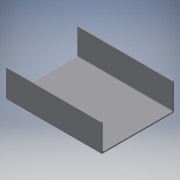
# Autodesk Inventor part: improved lift c chanel
Saved by Autodesk Inventor 2017 (Build 210142000, 142)
## iProperties
Created: 2019-02-04
Part Number: improved lift c chanel
Material: Generic
Document SubType Name: Modeling
Designer: S346852600
Density: 1 g/cm^3
Appearance: Default
Author: S346852600
Autodesk Inventor part; units mm, degrees
ref_plane "YZ Plane" through (0, 0, 0) normal (1, 0, 0) x (0, 1, 0)
ref_plane "XZ Plane" through (0, 0, 0) normal (0, 1, 0) x (-1, 0, 0)
ref_plane "XY Plane" through (0, 0, 0) normal (0, 0, 1) x (1, 0, 0)
sketch "Sketch1" plane through (0, 0, 0) normal (1, 0, 0) x (0, 1, 0)
  line L0 (0, 0) -> (-50.8, 0)
  line L1 (-53.975, -3.175) -> (-53.975, -161.925)
  line L2 (-50.8, -165.1) -> (0, -165.1)
  line L3 (0, -161.925) -> (-47.625, -161.925)
  line L4 (-50.8, -158.75) -> (-50.8, -6.35)
  line L5 (-47.625, -3.175) -> (0, -3.175)
  line L6 (0, 0) -> (0, -3.175)
  line L7 (0, -161.925) -> (0, -165.1)
  arc A0 (-50.8, 0) -> (-53.975, -3.175) centre (-50.8, -3.175) ccw
  arc A1 (-53.975, -161.925) -> (-50.8, -165.1) centre (-50.8, -161.925) ccw
  arc A2 (-47.625, -3.175) -> (-50.8, -6.35) centre (-47.625, -6.35) ccw
  arc A3 (-50.8, -158.75) -> (-47.625, -161.925) centre (-47.625, -158.75) ccw
  point P0 (-50.8, -161.925)
  point P1 (-50.8, -3.175)
  dimension "d3" = 3.175
  dimension "d4" = 50.8
  dimension "d5" = 158.75
  dimension "d6" = 3.175
  constraints: 16 end point, 8 point on circle, 8 tangent, 4 centre point, 4 perpendicular, 4 point on line, 3 equal radius, 2 collinear, 1 horizontal, 1 vertical, 2 other
  measures "d3" distance between parallel lines of L1 L4
  measures "d4" distance of point (-50.8, -3.175) L5.end
  measures "d5" distance of point (-50.8, -161.925) point (-50.8, -3.175)
  measures "d6" radius of A0
extrude "Extrusion1" add sketch "Sketch1" along normal blind 228.6
body "Solid1"
